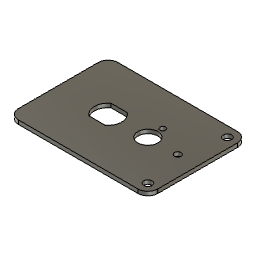
040036-01 Power Cord Plate (Autodesk Fusion 360 design; units mm, degrees)
Autodesk Fusion 360 part; units mm, degrees
note: some values were not read from the file. Chosen so that the rebuilt part matches the saved one: a side.
sketch "Sketch1" plane through (0, 0, 0) normal (0, 0, 1) x (1, 0, 0)
  line L0 (38.1, 31.75) -> (-38.1, 31.75)
  line L1 (-44.45, 25.4) -> (-44.45, -25.4)
  line L2 (-38.1, -31.75) -> (38.1, -31.75)
  line L3 (44.45, -25.4) -> (44.45, 25.4)
  line L4 (44.45, 31.75) -> (-44.45, -31.75) construction
  line L5 (-44.45, 31.75) -> (44.45, -31.75) construction
  circle A0 centre (38.1, 25.4) radius 2.625
  circle A1 centre (38.1, -25.4) radius 2.625
  line L6 (-44.45, 0) -> (44.45, 0) construction
  circle A2 centre (31.75, 0) radius 2.0955
  circle A3 centre (12.7, 0) radius 6.35
  circle A4 centre (12.7, 9.525) radius 1.7859
  line L7 (-17.8662, 7) -> (-7.5338, 7)
  line L8 (-7.5338, -7) -> (-17.8662, -7)
  arc A5 (-17.8662, 7) -> (-17.8662, -7) centre (-12.7, 0) ccw
  arc A6 (-7.5338, -7) -> (-7.5338, 7) centre (-12.7, 0) ccw
  line L9 (12.7, 9.525) -> (12.7, 0) construction
  arc A7 (-38.1, 31.75) -> (-44.45, 25.4) centre (-38.1, 25.4) ccw
  arc A8 (44.45, 25.4) -> (38.1, 31.75) centre (38.1, 25.4) ccw
  arc A9 (-44.45, -25.4) -> (-38.1, -31.75) centre (-38.1, -25.4) ccw
  arc A10 (38.1, -31.75) -> (44.45, -25.4) centre (38.1, -25.4) ccw
  dimension "d1" = 88.9
  dimension "d2" = 63.5
  dimension "d3" = 6.35
  dimension "d4" = 6.35
  dimension "d5" = 6.35
  dimension "d6" = 6.35
  dimension "d7" = 5.25
  dimension "d8" = 8.7
  dimension "d11" = 14
  dimension "d12" = 31.75
  dimension "d13" = 12.7
  dimension "d14" = 3.5719
  dimension "d16" = 9.525
  dimension "d17" = 12.7
  dimension "d18" = 4.191
  dimension "d19" = 31.75
  dimension "d20" = 6.35
  constraint horizontal L0
  constraint perpendicular L0 L1
  constraint parallel L0 L2
  constraint parallel L1 L3
  constraint coincident L4 origin
  constraint coincident L5 origin
  constraint equal A0 A1
  constraint coincident L6 A2.centre
  constraint coincident L6 A3.centre
  constraint coincident L6 A5.centre
  constraint horizontal L7
  constraint horizontal L8
  constraint coincident L8.start A5
  constraint concentric A5 A6
  constraint equal L7 L8
  constraint coincident A4.centre L9.start
  constraint coincident A3.centre L9.end
  constraint perpendicular L6 L9
  constraint coincident L1 L6.start
  constraint coincident L5.start L1
  constraint coincident L5.start L0
  constraint tangent L1 A7
  constraint tangent L0 A7
  constraint coincident L3 L6.end
  constraint coincident L4.start L0
  constraint coincident L4.start L3
  constraint tangent L0 A8
  constraint tangent L3 A8
  constraint coincident L4.end L1
  constraint coincident L4.end L2
  constraint tangent L1 A9
  constraint tangent L2 A9
  constraint coincident L5.end L2
  constraint coincident L5.end L3
  constraint tangent L2 A10
  constraint tangent L3 A10
  constraint midpoint L6 origin
  constraint equal A7 A8
  constraint equal A8 A10
  constraint equal A9 A10
  constraint horizontal L6
  measures "d1" distance of L4.end L5.end
  measures "d2" distance of L5.start L4.end
  measures "d3" distance of L3 A0.centre
  measures "d4" distance of L0 A0.centre
  measures "d5" distance of L3 A1.centre
  measures "d6" distance of L2 A1.centre
  measures "d7" diameter of A0
  measures "d8" radius of A5
  measures "d11" distance of L7 L8
  measures "d12" distance of L1 A5.centre
  measures "d13" diameter of A3
  measures "d14" diameter of A4
  measures "d16" distance of A4.centre A3.centre
  measures "d17" distance of L3 A2.centre
  measures "d18" diameter of A2
  measures "d19" distance of L3 A3.centre
  measures "d20" radius of A7
extrude "Face1" add sketch "Sketch1" against normal blind 2.5
equation "d3 = MountingHoleOffset"
equation "d4 = MountingHoleOffset"
equation "d5 = MountingHoleOffset"
equation "d6 = MountingHoleOffset"
equation "d7 = MountingHole"
equation "d8 = StrainReliefRadius"
equation "d11 = StrainReliefFlatWidth"
equation "d12 = 1 1/4\""
equation "d13 = PowerSwitchHole"
equation "d14 = PowerSwitchLocatorHole"
equation "d16 = PowerSwitchLocatorOffset"
equation "d17 = ( 1 / 2 ) * 1 in"
equation "d18 = ThreadedStudMountingHole"
equation "d19 = 1 1/4\""
equation "d20 = CornerRadius"
equation "MountingHoleOffset = ( 1 / 4 ) * 1 in"
equation "CornerRadius = ( 1 / 4 ) * 1 in"
equation "PowerSwitchHole = ( 1 / 2 ) * 1 in"
equation "PowerSwitchLocatorHole = ( 9 / 64 ) * 1 in"
equation "PowerSwitchLocatorOffset = ( 3 / 8 ) * 1 in"
equation "ThreadedStudMountingHole = 0.165 in"
equation "MountingHole = 5.25 mm"
equation "StrainReliefFlatWidth = 14 mm"
equation "StrainReliefRadius = 17.4 mm / 2"
